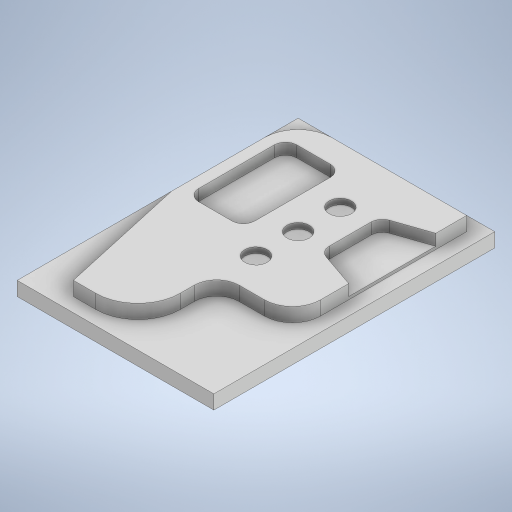
# Autodesk Inventor part: Exercise4
Saved by Autodesk Inventor 2023 (Build 270158000, 158)
## iProperties
Created: 2023-04-25
Part Number: Exercise4
Material: Generic
Document SubType Name: Modeling
Designer: dell
Density: 1 g/cm^3
Appearance: Default
Author: dell
Autodesk Inventor part; units mm, degrees
ref_plane "YZ Plane" through (0, 0, 0) normal (1, 0, 0) x (0, 1, 0)
ref_plane "XZ Plane" through (0, 0, 0) normal (0, 1, 0) x (-1, 0, 0)
ref_plane "XY Plane" through (0, 0, 0) normal (0, 0, 1) x (1, 0, 0)
sketch "Sketch1" plane through (0, 0, 0) normal (0, 1, 0) x (-1, 0, 0)
  line L0 (35, 50) -> (-35, 50)
  line L1 (-35, 50) -> (-35, -50)
  line L2 (-35, -50) -> (35, -50)
  line L3 (35, -50) -> (35, 50)
  line L4 (35, 50) -> (-35, -50) construction
  line L5 (-35, 50) -> (35, -50) construction
  point P0 (0, 0)
  dimension "d0" = 100
  dimension "d1" = 70
  constraints: 12 end point, 2 midpoint, 2 parallel, 1 horizontal, 1 perpendicular
  measures "d0" distance of L2.end L0.start
  measures "d1" distance of L1.end L2.end
extrude "Extrusion1" add sketch "Sketch1" along normal blind 5
sketch "Sketch2" plane through (0, 5, 0) normal (0, 1, 0) x (1, 0, 0)
  line L0 (30, 45) -> (30, -7)
  line L1 (-18, 45) -> (30, 45)
  line L2 (-35, -50) -> (35, -50) projected
  line L3 (35, -50) -> (35, 50) projected
  arc A0 (-18, 45) -> (-30, 33) centre (-18, 33) ccw
  line L4 (-30, 33) -> (-30, 0)
  line L5 (-30, 0) -> (-20, -45)
  arc A1 (-12, -45) -> (3, -30) centre (-12, -30) ccw
  line L6 (-20, -45) -> (-12, -45)
  line L7 (3, -30) -> (3, -25)
  arc A2 (11, -17) -> (3, -25) centre (11, -25) ccw
  arc A3 (20, -17) -> (30, -7) centre (20, -7) ccw
  line L8 (11, -17) -> (20, -17)
  point P0 (0, 0)
  dimension "d4" = 95
  dimension "d5" = 5
  dimension "d6" = 24
  dimension "d7" = 65
  dimension "d8" = 50
  dimension "d9" = 55
  dimension "d10" = 5
  dimension "d11" = 30
  dimension "d12" = 32
  dimension "d13" = 16
  dimension "d15" = 20
  constraints: 14 end point, 8 point on circle, 8 tangent, 4 centre point, 3 vertical, 1 horizontal, 1 perpendicular
  measures "d4" distance between parallel lines of L2 L1
  measures "d5" distance between parallel lines of L3 L0
  measures "d6" diameter of A0
  measures "d7" distance between parallel lines of L3 L4
  measures "d8" distance from line of L2 L4.end
  measures "d9" distance from line of L3 L5.end
  measures "d10" distance from line of L2 L5.end
  measures "d11" diameter of A1
  measures "d12" distance between parallel lines of L3 L7
  measures "d13" diameter of A2
  measures "d15" diameter of A3
extrude "Extrusion2" add sketch "Sketch2" along normal blind 5
sketch "Sketch3" plane through (0, 10, 0) normal (0, 1, 0) x (1, 0, 0)
  line L0 (-22, 1.52) -> (-10, 1.52)
  line L1 (-6, 5.52) -> (-6, 32.52)
  line L2 (-10, 36.52) -> (-22, 36.52)
  line L3 (-26, 32.52) -> (-26, 5.52)
  line L4 (-23.2444, 1.52) -> (-8.7556, 34.48) construction
  line L5 (-6.9662, 2.9131) -> (-22.5304, 28.9061) construction
  arc A0 (-6, 32.52) -> (-10, 36.52) centre (-10, 32.52) ccw
  arc A1 (-22, 36.52) -> (-26, 32.52) centre (-22, 32.52) ccw
  arc A2 (-26, 5.52) -> (-22, 1.52) centre (-22, 5.52) ccw
  arc A3 (-10, 1.52) -> (-6, 5.52) centre (-10, 5.52) ccw
  line L6 (35, -50) -> (35, 50) projected
  line L7 (-35, -50) -> (35, -50) projected
  line L8 (15, 26) -> (15, 11)
  line L9 (30, 7) -> (30, 30)
  line L10 (30, 30) -> (15, 7) construction
  line L11 (15, 30) -> (30, 7) construction
  line L12 (30, -7) -> (30, 45) projected
  arc A4 (19, 30) -> (15, 26) centre (19, 26) ccw
  arc A5 (15, 11) -> (19, 7) centre (19, 11) ccw
  line L13 (30, 34) -> (17.7027, 29.7838)
  line L14 (30, 3) -> (17.7027, 7.2162)
  line L15 (30, 7) -> (30, 3)
  line L16 (30, 34) -> (30, 30)
  point P0 (0, 0)
  point P1 (-16, 18)
  point P2 (-26, 19.02)
  point P3 (-16, 36.52)
  point P4 (22.5, 18.5)
  point P5 (22.5, 7)
  dimension "d18" = 8
  dimension "d19" = 8
  dimension "d20" = 8
  dimension "d22" = 8
  dimension "d23" = 35
  dimension "d24" = 20
  dimension "d25" = 51
  dimension "d26" = 68
  dimension "d27" = 51
  dimension "d28" = 20
  dimension "d29" = 0
  dimension "d32" = 8
  dimension "d33" = 8
  dimension "d34" = 84
  dimension "d35" = 53
  constraints: 28 end point, 15 point on circle, 12 tangent, 6 centre point, 5 midpoint, 3 parallel, 3 point on line, 1 collinear, 1 horizontal, 1 perpendicular
  measures "d18" diameter of A2
  measures "d19" diameter of A1
  measures "d20" diameter of A0
  measures "d22" diameter of A3
  measures "d23" distance between parallel lines of L0 L2
  measures "d24" distance from line of L1 point (-26, 19.02)
  measures "d25" distance from line of L6 point (-16, 36.52)
  measures "d26" distance from line of L7 point (-16, 18)
  measures "d27" distance from line of L6 point (-16, 18)
  measures "d28" distance between parallel lines of L6 L8
  measures "d29" distance between parallel lines of L12 L9
  measures "d32" diameter of A4
  measures "d33" diameter of A5
  measures "d34" distance from line of L7 L13.start
  measures "d35" distance from line of L7 L14.start
extrude "Extrusion3" cut sketch "Sketch3" against normal blind 4
sketch "Sketch4" plane through (0, 10, 0) normal (0, 1, 0) x (1, 0, 0)
  circle A0 centre (5, -5) radius 4
  circle A1 centre (5, 10) radius 4
  circle A2 centre (5, 25) radius 4
  line L0 (-35, -50) -> (35, -50) projected
  line L1 (35, -50) -> (35, 50) projected
  point P0 (0, 0)
  dimension "d38" = 8
  dimension "d39" = 8
  dimension "d40" = 8
  dimension "d41" = 45
  dimension "d42" = 60
  dimension "d43" = 75
  dimension "d44" = 30
  dimension "d45" = 30
  dimension "d46" = 30
  constraints: 3 centre point
  measures "d38" diameter of A2
  measures "d39" diameter of A1
  measures "d40" diameter of A0
  measures "d41" distance from line of L0 A0.centre
  measures "d42" distance from line of L0 A1.centre
  measures "d43" distance from line of L0 A2.centre
  measures "d44" distance from line of L1 A2.centre
  measures "d45" distance from line of L1 A1.centre
  measures "d46" distance from line of L1 A0.centre
extrude "Extrusion4" cut sketch "Sketch4" against normal blind 2
body "Solid1"
